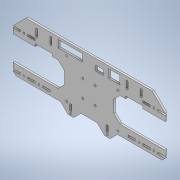
# Autodesk Inventor part: Деталь3
Saved by Autodesk Inventor 2020 (Build 240168000, 168)
## iProperties
Created: 2025-01-24
Part Number: Деталь3
Material: Типовые
Document SubType Name: Modeling
Designer: frozj
Density: 1 g/cm^3
Appearance: По умолчанию
Author: frozj
Autodesk Inventor part; units mm, degrees
ref_plane "YZ Plane" through (0, 0, 0) normal (1, 0, 0) x (0, 1, 0)
ref_plane "XZ Plane" through (0, 0, 0) normal (0, 1, 0) x (-1, 0, 0)
ref_plane "XY Plane" through (0, 0, 0) normal (0, 0, 1) x (1, 0, 0)
sketch "Эскиз1" plane through (0, 0, 0) normal (0, 0, 1) x (1, 0, 0)
  line L0 (123, -10) -> (-123, -10)
  line L1 (-123, -10) -> (-123, 10)
  line L2 (-123, 10) -> (123, 10)
  line L3 (123, 10) -> (123, -10)
  line L4 (123, -28.5) -> (-123, -28.5)
  line L5 (-123, -28.5) -> (-123, 28.5)
  line L6 (-123, 28.5) -> (123, 28.5)
  line L7 (123, 28.5) -> (123, -28.5)
  line L8 (123, -28.5) -> (-123, 28.5) construction
  line L9 (-123, -28.5) -> (123, 28.5) construction
  line L10 (10, -14) -> (-10, -14)
  line L11 (-10, -14) -> (-10, 14)
  line L12 (-10, 14) -> (10, 14)
  line L13 (10, 14) -> (10, -14)
  circle A0 centre (-10, 14) radius 1.5
  line L14 (0, 4.14) -> (0, 0)
  line L15 (0, 0) -> (3.9539, 0)
  circle A1 centre (10, 14) radius 1.5
  circle A2 centre (-10, -14) radius 1.5
  circle A3 centre (10, -14) radius 1.5
  line L16 (-123, -20) -> (-40, -20)
  line L17 (-40, -20) -> (-40, 20)
  line L18 (-40, 20) -> (-123, 20)
  line L19 (-123, 20) -> (-123, -20)
  line L20 (-40, -20) -> (-50, -20)
  line L21 (-50, -20) -> (-50, 20)
  line L22 (-50, 20) -> (-40, 20)
  line L23 (-40, 20) -> (-40, -20)
  line L24 (-50, 10) -> (-96, 10)
  line L25 (-96, 10) -> (-96, -10)
  line L26 (-96, -10) -> (-50, -10)
  line L27 (-50, -10) -> (-50, 10)
  line L28 (-50, 20) -> (-40, 10)
  line L29 (-40, -10) -> (-50, -20)
  line L30 (50, -35) -> (-50, -35)
  line L31 (-50, -35) -> (-50, 35)
  line L32 (-50, 35) -> (50, 35)
  line L33 (50, 35) -> (50, -35)
  line L34 (50, -35) -> (-50, 35) construction
  line L35 (-50, -35) -> (50, 35) construction
  line L36 (123, -20) -> (40, -20)
  line L37 (40, -20) -> (40, 20)
  line L38 (40, 20) -> (123, 20)
  line L39 (50, 20) -> (40, 10)
  line L40 (40, -10) -> (50, -20)
  line L41 (-50, -35) -> (-36, -35)
  line L42 (-50, -31) -> (-50, -35)
  circle A4 centre (-36, -31) radius 1.5
  line L43 (-50, 35) -> (-36, 35)
  line L44 (-50, 32.5) -> (-50, 35)
  circle A5 centre (-36, 32.5) radius 1.5
  line L45 (50, -35) -> (47, -35)
  line L46 (50, -31) -> (50, -35)
  circle A6 centre (47, -31) radius 1.5
  line L47 (50, 35) -> (47, 35)
  line L48 (50, 26) -> (50, 35)
  circle A7 centre (47, 26) radius 1.5
  line L49 (-123, 28.5) -> (123, 28.5)
  line L50 (123, 28.5) -> (123, 31.5)
  line L51 (123, 31.5) -> (-123, 31.5)
  line L52 (-123, 31.5) -> (-123, 28.5)
  line L53 (-123, -28.5) -> (123, -28.5)
  line L54 (123, -28.5) -> (123, -31.5)
  line L55 (123, -31.5) -> (-123, -31.5)
  line L56 (-123, -31.5) -> (-123, -28.5)
  line L57 (-123, 31.5) -> (-111, 31.5)
  line L58 (-111, 31.5) -> (-111, 28.5)
  line L59 (-111, 28.5) -> (-123, 28.5)
  line L60 (-123, 28.5) -> (-123, 31.5)
  line L61 (-111, 28.5) -> (-99, 28.5)
  line L62 (-99, 28.5) -> (-99, 31.5)
  line L63 (-99, 31.5) -> (-111, 31.5)
  line L64 (-111, 31.5) -> (-111, 28.5)
  circle A8 centre (-105, 30) radius 1.5
  line L65 (-99, 28.5) -> (-87, 28.5)
  line L66 (-87, 28.5) -> (-87, 31.5)
  line L67 (-87, 31.5) -> (-99, 31.5)
  line L68 (-99, 31.5) -> (-99, 28.5)
  line L69 (-87, 28.5) -> (-59, 28.5)
  line L70 (-59, 28.5) -> (-59, 52.5)
  line L71 (-59, 52.5) -> (-87, 52.5)
  line L72 (-87, 52.5) -> (-87, 28.5)
  line L73 (-87, 52.5) -> (-79, 52.5)
  line L74 (-79, 52.5) -> (-79, 28.5)
  line L75 (-79, 28.5) -> (-87, 28.5)
  line L76 (-87, 28.5) -> (-87, 52.5)
  line L77 (-59, 52.5) -> (-67, 52.5)
  line L78 (-67, 52.5) -> (-67, 28.5)
  line L79 (-67, 28.5) -> (-59, 28.5)
  line L80 (-59, 28.5) -> (-59, 52.5)
  line L81 (-59, 52.5) -> (-61.5, 52.5)
  line L82 (-59, 45.5) -> (-59, 52.5)
  circle A9 centre (-61.5, 45.5) radius 1.5
  line L83 (-59, 28.5) -> (-61.5, 28.5)
  line L84 (-59, 35.5) -> (-59, 28.5)
  circle A10 centre (-61.5, 35.5) radius 1.5
  line L85 (-63, 45.5) -> (-63, 35.5)
  line L86 (-60, 35.5) -> (-60, 45.5)
  line L87 (-73, 40.5) -> (-73, 52.5)
  circle A11 centre (-84.5, 45.5) radius 1.5
  circle A12 centre (-84.5, 35.5) radius 1.5
  line L88 (-83, 45.5) -> (-83, 35.5)
  line L89 (-86, 35.5) -> (-86, 45.5)
  line L90 (123, 28.5) -> (-123, 28.5)
  line L91 (59, 28.5) -> (59, 52.5)
  line L92 (59, 52.5) -> (87, 52.5)
  line L93 (87, 52.5) -> (87, 28.5)
  line L94 (87, 52.5) -> (79, 52.5)
  line L95 (79, 52.5) -> (79, 28.5)
  line L96 (67, 52.5) -> (67, 28.5)
  line L97 (59, 45.5) -> (59, 52.5)
  circle A13 centre (61.5, 45.5) radius 1.5
  circle A14 centre (61.5, 35.5) radius 1.5
  line L98 (63, 45.5) -> (63, 35.5)
  line L99 (60, 35.5) -> (60, 45.5)
  line L100 (83, 45.5) -> (83, 35.5)
  circle A15 centre (84.5, 45.5) radius 1.5
  line L101 (86, 35.5) -> (86, 45.5)
  circle A16 centre (84.5, 35.5) radius 1.5
  line L102 (-123, 31.5) -> (123, 31.5)
  line L103 (123, 31.5) -> (123, 52.5)
  line L104 (123, 52.5) -> (-123, 52.5)
  line L105 (-123, 52.5) -> (-123, 31.5)
  line L106 (111, 31.5) -> (111, 28.5)
  line L107 (99, 28.5) -> (99, 31.5)
  circle A17 centre (105, 30) radius 1.5
  line L108 (99, 31.5) -> (99, 28.5)
  line L109 (-123, -28.5) -> (-111, -28.5)
  line L110 (-111, -28.5) -> (-111, -31.5)
  line L111 (-111, -31.5) -> (-123, -31.5)
  line L112 (-123, -31.5) -> (-123, -28.5)
  line L113 (-111, -31.5) -> (-99, -31.5)
  line L114 (-99, -31.5) -> (-99, -28.5)
  line L115 (-99, -28.5) -> (-111, -28.5)
  line L116 (-111, -28.5) -> (-111, -31.5)
  circle A18 centre (-105, -30) radius 1.5
  line L117 (-99, -28.5) -> (-87, -28.5)
  line L118 (-87, -28.5) -> (-87, -31.5)
  line L119 (-87, -31.5) -> (-99, -31.5)
  line L120 (-99, -31.5) -> (-99, -28.5)
  line L121 (-87, -31.5) -> (-75, -31.5)
  line L122 (-75, -31.5) -> (-75, -28.5)
  line L123 (-75, -28.5) -> (-87, -28.5)
  line L124 (-87, -28.5) -> (-87, -31.5)
  circle A19 centre (-81, -30) radius 1.5
  line L125 (111, -28.5) -> (111, -31.5)
  line L126 (99, -31.5) -> (99, -28.5)
  circle A20 centre (105, -30) radius 1.5
  line L127 (75, -31.5) -> (75, -28.5)
  line L128 (87, -28.5) -> (87, -31.5)
  circle A21 centre (81, -30) radius 1.5
  line L129 (-123, -31.5) -> (123, -31.5)
  line L130 (123, -31.5) -> (123, -36.5)
  line L131 (123, -36.5) -> (-123, -36.5)
  line L132 (-123, -36.5) -> (-123, -31.5)
  line L133 (-123, -36.5) -> (123, -36.5)
  line L134 (123, -36.5) -> (123, -48.5)
  line L135 (123, -48.5) -> (-123, -48.5)
  line L136 (-123, -48.5) -> (-123, -36.5)
  line L137 (0, -36.5) -> (-29.5, -36.5)
  line L138 (-29.5, -48.5) -> (0, -48.5)
  line L139 (0, -48.5) -> (0, -36.5)
  line L140 (-29.5, -48.5) -> (-28, -48.5)
  line L141 (-28, -48.5) -> (-28, -41.5)
  line L142 (-28, -41.5) -> (-29.5, -41.5)
  line L143 (-29.5, -48.5) -> (-31, -48.5)
  line L144 (-31, -48.5) -> (-31, -41.5)
  line L145 (-31, -41.5) -> (-29.5, -41.5)
  circle A22 centre (-29.5, -45) radius 1.5
  line L146 (-28, -41.5) -> (-31, -41.5)
  line L147 (-31, -41.5) -> (-31, -31.5)
  line L148 (-31, -31.5) -> (-28, -31.5)
  line L149 (-28, -31.5) -> (-28, -41.5)
  line L150 (28, -41.5) -> (29.5, -41.5)
  circle A23 centre (29.5, -45) radius 1.5
  line L151 (28, -41.5) -> (31, -41.5)
  line L152 (31, -41.5) -> (31, -31.5)
  line L153 (31, -31.5) -> (28, -31.5)
  line L154 (28, -31.5) -> (28, -41.5)
  line L155 (-28, -48.5) -> (-25, -48.5)
  line L156 (-25, -48.5) -> (-13, -36.5)
  line L157 (-31, -48.5) -> (-34, -48.5)
  line L158 (-34, -48.5) -> (-46, -36.5)
  line L159 (25, -48.5) -> (13, -36.5)
  line L160 (34, -48.5) -> (46, -36.5)
  line L161 (-75, -31.5) -> (-63, -31.5)
  line L162 (-63, -31.5) -> (-63, -28.5)
  line L163 (-63, -28.5) -> (-75, -28.5)
  line L164 (-75, -28.5) -> (-75, -31.5)
  line L165 (75, -31.5) -> (63, -31.5)
  line L166 (63, -31.5) -> (63, -28.5)
  line L167 (63, -28.5) -> (75, -28.5)
  line L168 (75, -28.5) -> (75, -31.5)
  line L169 (59, 28.5) -> (87, 28.5)
  line L170 (87, 28.5) -> (87, 20)
  line L171 (87, 20) -> (59, 20)
  line L172 (59, 20) -> (59, 28.5)
  line L173 (87, 20) -> (59, 20)
  line L174 (59, 20) -> (59, 24)
  line L175 (59, 24) -> (87, 24)
  line L176 (87, 24) -> (87, 20)
  line L177 (-59, 20) -> (-59, 24)
  line L178 (-59, 24) -> (-87, 24)
  line L179 (-87, 24) -> (-87, 20)
  line L180 (50, 35) -> (31.5, 35)
  line L181 (31.5, 35) -> (31.5, 48.5)
  line L182 (31.5, 48.5) -> (50, 48.5)
  line L183 (50, 48.5) -> (50, 35)
  line L184 (31.5, 35) -> (23.5, 35)
  line L185 (23.5, 35) -> (23.5, 48.5)
  line L186 (23.5, 48.5) -> (31.5, 48.5)
  line L187 (31.5, 48.5) -> (31.5, 35)
  line L188 (23.5, 35) -> (10.5, 35)
  line L189 (10.5, 35) -> (10.5, 43)
  line L190 (10.5, 43) -> (23.5, 43)
  line L191 (23.5, 43) -> (23.5, 35)
  line L192 (10.5, 35) -> (-10.5, 35)
  line L193 (-10.5, 35) -> (-10.5, 48.5)
  line L194 (-10.5, 48.5) -> (10.5, 48.5)
  line L195 (10.5, 48.5) -> (10.5, 35)
  line L196 (-10.5, 48.5) -> (-50, 48.5)
  line L197 (-50, 48.5) -> (-50, 35)
  line L198 (-50, 35) -> (-10.5, 35)
  line L199 (-10.5, 35) -> (-10.5, 48.5)
  line L200 (-50, 35) -> (-10.5, 35)
  line L201 (-10.5, 35) -> (-10.5, 37)
  line L202 (-10.5, 37) -> (-50, 37)
  line L203 (-50, 37) -> (-50, 35)
  line L204 (-123, -31.5) -> (-118, -36.5)
  line L205 (123, -31.5) -> (118, -36.5)
  line L206 (123, 31.5) -> (102, 52.5)
  line L207 (-123, 31.5) -> (-102, 52.5)
  point P0 (0, 0)
  point P1 (-40, -10)
  point P2 (-123, -31.5)
  point P3 (-34.882, 31.5)
  point P4 (-37.118, 31.5)
  point P5 (87, 31.5)
  point P6 (-31, -45)
  point P7 (-28, -45)
  point P8 (105, -28.5)
  point P9 (105, -31.5)
  point P10 (81, -31.5)
  point P11 (81, -28.5)
  point P12 (-123, -31.5)
  dimension "d0" = 246
  dimension "d1" = 20
  dimension "d3" = 123
  dimension "d4" = 57
  dimension "d5" = 20
  dimension "d6" = 28
  dimension "d7" = 3
  dimension "d10" = 10
  dimension "d11" = 246
  dimension "d12" = 10
  dimension "d13" = 14
  dimension "d14" = 83
  dimension "d15" = 40
  dimension "d16" = 20
  dimension "d17" = 10
  dimension "d18" = 46
  dimension "d19" = 100
  dimension "d20" = 70
  dimension "d23" = 3
  dimension "d24" = 36
  dimension "d25" = 31
  dimension "d26" = 50
  dimension "d27" = 35
  dimension "d30" = 3
  dimension "d31" = 2.5
  dimension "d32" = 14
  dimension "d35" = 3
  dimension "d39" = 3
  dimension "d40" = 4
  dimension "d41" = 3
  dimension "d42" = 2.5
  dimension "d43" = 3
  dimension "d44" = 3
  dimension "d45" = 3
  dimension "d46" = 12
  dimension "d47" = 12
  dimension "d48" = 3
  dimension "d50" = 1.5
  dimension "d51" = 6
  dimension "d52" = 12
  dimension "d53" = 28
  dimension "d54" = 24
  dimension "d55" = 8
  dimension "d56" = 8
  dimension "d59" = 3
  dimension "d60" = 2.5
  dimension "d61" = 7
  dimension "d64" = 3
  dimension "d67" = 2.5
  dimension "d69" = 7
  dimension "d70" = 12
  dimension "d71" = 12
  dimension "d72" = 12
  dimension "d73" = 12
  dimension "d74" = 5
  dimension "d75" = 246
  dimension "d76" = 12
  dimension "d77" = 1.5
  dimension "d78" = 1.5
  dimension "d79" = 6
  dimension "d80" = 3
  dimension "d81" = 6
  dimension "d82" = 3
  dimension "d83" = 29.5
  constraints: 414 end point, 70 symmetric about line, 68 parallel, 44 horizontal, 38 perpendicular, 34 point on line, 24 centre point, 16 point on circle, 6 midpoint, 3 tangent, 1 coincident, 1 vertical, 18 other
  measures "d0" distance of L1.end L2.end
  measures "d1" distance of L0.end L1.end
  measures "d3" distance from line of L3 point (0, 0)
  measures "d4" distance of L4.end L5.end
  measures "d5" distance of L11.end L12.end
  measures "d6" distance of L10.end L11.end
  measures "d7" diameter of A0
  measures "d10" distance from line of L2 point (0, 0)
  measures "d11" distance between parallel lines of L5 L7
  measures "d12" distance from line of point (0, 0) L13
  measures "d13" distance from line of L12 point (0, 0)
  measures "d14" distance of L18.end L17.end
  measures "d15" distance of L17.end L16.end
  measures "d16" distance from line of point (0, 0) L18
  measures "d17" distance of L21.end L22.end
  measures "d18" distance of L26.end L25.end
  measures "d19" distance of L31.end L32.end
  measures "d20" distance of L30.end L31.end
  measures "d23" diameter of A4
  measures "d24" horizontal distance of point (0, 0) A4.centre
  measures "d25" vertical distance of A4.centre point (0, 0)
  measures "d26" distance from line of point (0, 0) L31
  measures "d27" distance from line of L30 point (0, 0)
  measures "d30" diameter of A5
  measures "d31" distance from line of L32 A5.centre
  measures "d32" distance from line of L31 A5.centre
  measures "d35" diameter of A6
  measures "d39" distance from line of A6.centre L33
  measures "d40" distance from line of L30 A6.centre
  measures "d41" distance from line of L33 A7.centre
  measures "d42" distance from line of L6 A7.centre
  measures "d43" diameter of A7
  measures "d44" distance of L50.end L49.end
  measures "d45" distance of L53.end L54.end
  measures "d46" distance of L58.end L59.end
  measures "d47" distance of L63.end L62.end
  measures "d48" diameter of A8
  measures "d50" distance from line of L51 A8.centre
  measures "d51" distance from line of L62 A8.centre
  measures "d52" distance of L67.end L66.end
  measures "d53" distance of L71.end L70.end
  measures "d54" distance of L70.end L69.end
  measures "d55" distance of L74.end L75.end
  measures "d56" distance of L79.end L78.end
  measures "d59" diameter of A9
  measures "d60" distance from line of A9.centre L70
  measures "d61" distance from line of L71 A9.centre
  measures "d64" diameter of A10
  measures "d67" distance from line of L84 A10.centre
  measures "d69" distance from line of L6 A10.centre
  measures "d70" distance of L110.end L111.end
  measures "d71" distance of L115.end L114.end
  measures "d72" distance of L118.end L119.end
  measures "d73" distance of L123.end L122.end
  measures "d74" distance of L129.end L130.end
  measures "d75" distance of L134.end L135.end
  measures "d76" distance of L133.end L134.end
  measures "d77" distance from line of L4 A18.centre
  measures "d78" distance from line of L4 A19.centre
  measures "d79" distance from line of L124 A19.centre
  measures "d80" diameter of A18
  measures "d81" distance from line of L120 A18.centre
  measures "d82" diameter of A19
  measures "d83" distance of L138.end L138.start
extrude "Выдавливание1" add sketch "Эскиз1" along normal blind 3 contours L17 L2 L11 L0 | L0 L11 A2 L10 A3 L13 L37 L36 L33 L4 L31 L16 L17 | L17 L16 L29 | L11 L2 L13 L0 | L0 L13 A3 L10 A2 L11 | L17 L18 L31 L6 L33 L38 L37 L2 L13 A1 L12 A0 L11 | L28 L18 L17 | L31 L4 L5 L16 | L13 L2 L37 L0 | L11 A0 L12 A1 L13 L2 | L18 L177 L178 L179 L5 L6 L31 | L31 L55 L162 L4 | L4 L33 L55 A6 A4 L31 | L40 L36 L37 | L31 L51 A5 L33 L6 | L6 L70 L51 L31 | L33 L36 L7 L4 | L4 L166 L55 L33 | L37 L38 L39 | L6 L78 L51 L70 | L33 L51 L91 L6 | L6 L172 L38 L33 | L51 L70 L104 L91 L33 L183 L182 L186 L185 L190 L195 L194 L196 L197 L31 | L31 L32 L33 L51 A5 | L4 A18 L55 L110 | L55 L31 L30 L147 L131 L204 | L122 L55 A19 L4 | L55 A4 L147 L30 L31 | L51 L78 L71 L70 | L91 L51 L96 L6 | L6 L170 L175 L172 | L4 L114 L55 A18 | L4 A21 L55 L127 | L55 L205 L131 L152 L30 L33 | L33 L30 L152 L55 A6 | A19 L55 L118 L4 | L6 L74 L51 L78 | L51 L74 L71 L78 | L96 L51 L95 L6 | L91 L92 L96 L51 | L197 L202 L193 L32 | L131 L147 L144 L135 L158 | L4 L128 L55 A21 | L58 L51 A8 L6 | L207 L104 L72 L51 | L38 L170 L6 L7 | L125 L55 A20 L4 | L6 L66 L51 L74 | L51 L72 L71 L74 | L95 L51 L93 L6 | L96 L92 L95 L51 | A8 L51 L62 L6 | A20 L55 L126 L4 | L95 L92 L93 L51 | L32 L185 L186 L181 | L193 L194 L195 L189 L32 | L144 A22 L141 L135 | L145 L142 L141 A22 L144 | L149 L55 L154 L30 | L30 L154 L131 L149 | L6 A17 L51 L106 | L51 L93 L104 L206 | L160 L135 L159 L131 L154 L150 L151 L152 | L107 L51 A17 L6 | L131 L156 L135 L141 L149
